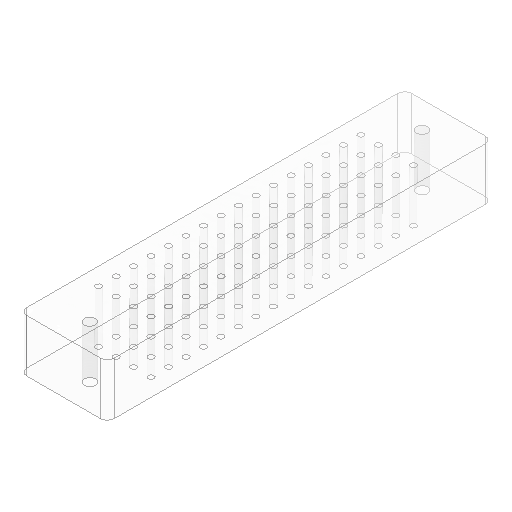
# Autodesk Inventor part: ICT-00-034
Saved by Autodesk Inventor 2026.1 (Build 301233020, 233B)
## iProperties
Company: Delta
Created: 2025-10-08
Part Number: ICT-00-034
Material: Acrílico TP
Document SubType Name: Modeling
Designer: Willian Pinheiro
Density: 1.19 g/cm^3
Appearance: Transparent - Clear
Description: Chapa T Agulha Auxiliar
Mass: 46.1991 g
Surface Area: 145.472 cm^2
Volume: 38.8228 cm^3
Dimensões: 15 x 25 x 110 mm
Total: 1
Author: Willian Pinheiro
Revision Number: 00
Title: ICT
Autodesk Inventor part; units mm, degrees
ref_plane "YZ Plane" through (0, 0, 0) normal (1, 0, 0) x (0, 1, 0)
ref_plane "XZ Plane" through (0, 0, 0) normal (0, 1, 0) x (-1, 0, 0)
ref_plane "XY Plane" through (0, 0, 0) normal (0, 0, 1) x (1, 0, 0)
sketch "Sketch1" plane through (0, 0, 0) normal (0, 0, 1) x (1, 0, 0)
  line L0 (-17.5, 0) -> (17.5, 0) construction
  line L1 (0, -77) -> (0, 77) construction
  line L2 (-12.5, 55) -> (12.5, 55)
  line L3 (12.5, 55) -> (12.5, -55)
  line L4 (12.5, -55) -> (-12.5, -55)
  line L5 (-12.5, -55) -> (-12.5, 55)
  line L6 (-7.5, -37.5) -> (7.5, -37.5) construction
  line L7 (7.5, -37.5) -> (7.5, 37.5) construction
  line L8 (7.5, 37.5) -> (-7.5, 37.5) construction
  line L9 (-7.5, 37.5) -> (-7.5, -37.5) construction
  line L10 (0, 37.5) -> (0, -37.5) construction
  circle A0 centre (0, -47.5) radius 4
  line L11 (-10.5, -40.5) -> (10.5, -40.5) construction
  line L12 (10.5, -40.5) -> (10.5, 40.5) construction
  line L13 (10.5, 40.5) -> (-10.5, 40.5) construction
  line L14 (-10.5, 40.5) -> (-10.5, -40.5) construction
  point P0 (0, 0)
  point P1 (-7.5, -32.5)
  point P2 (-7.5, -27.5)
  point P3 (-7.5, -22.5)
  point P4 (-7.5, -17.5)
  point P5 (-7.5, -12.5)
  point P6 (-7.5, -7.5)
  point P7 (-7.5, -2.5)
  point P8 (-7.5, 2.5)
  point P9 (-7.5, 7.5)
  point P10 (-7.5, 12.5)
  point P11 (-7.5, 17.5)
  point P12 (-7.5, 22.5)
  point P13 (-7.5, 27.5)
  point P14 (-7.5, 32.5)
  point P15 (-2.5, -37.5)
  point P16 (-2.5, -32.5)
  point P17 (-2.5, -27.5)
  point P18 (-2.5, -22.5)
  point P19 (-2.5, -17.5)
  point P20 (-2.5, -12.5)
  point P21 (-2.5, -7.5)
  point P22 (-2.5, -2.5)
  point P23 (-2.5, 2.5)
  point P24 (-2.5, 7.5)
  point P25 (-2.5, 12.5)
  point P26 (-2.5, 17.5)
  point P27 (-2.5, 22.5)
  point P28 (-2.5, 27.5)
  point P29 (-2.5, 32.5)
  point P30 (-2.5, 37.5)
  point P31 (2.5, -37.5)
  point P32 (2.5, -32.5)
  point P33 (2.5, -27.5)
  point P34 (2.5, -22.5)
  point P35 (2.5, -17.5)
  point P36 (2.5, -12.5)
  point P37 (2.5, -7.5)
  point P38 (2.5, -2.5)
  point P39 (2.5, 2.5)
  point P40 (2.5, 7.5)
  point P41 (2.5, 12.5)
  point P42 (2.5, 17.5)
  point P43 (2.5, 22.5)
  point P44 (2.5, 27.5)
  point P45 (2.5, 32.5)
  point P46 (2.5, 37.5)
  point P47 (7.5, -32.5)
  point P48 (7.5, -27.5)
  point P49 (7.5, -22.5)
  point P50 (7.5, -17.5)
  point P51 (7.5, -12.5)
  point P52 (7.5, -7.5)
  point P53 (7.5, -2.5)
  point P54 (7.5, 2.5)
  point P55 (7.5, 7.5)
  point P56 (7.5, 12.5)
  point P57 (7.5, 17.5)
  point P58 (7.5, 22.5)
  point P59 (7.5, 27.5)
  point P60 (7.5, 32.5)
  point P61 (0, 47.5)
  dimension "d0" = 110
  dimension "d1" = 25
  dimension "d4" = 5
  dimension "d7" = 5
  dimension "d19" = 7.5
  dimension "d20" = 8
  dimension "d21" = 3
  dimension "d22" = 81
  dimension "d23" = 21
  constraints: 26 end point, 6 parallel, 3 horizontal, 3 perpendicular, 2 midpoint, 1 centre point, 1 coincident, 1 point on line, 1 symmetric about line, 1 vertical, 70 other
  measures "d0" distance of L4.end L2.start
  measures "d1" distance of L2.start L2.end
  measures "d4" distance of L6.start point (-7.5, -32.5)
  measures "d7" distance of L6.start point (-2.5, -37.5)
  measures "d19" distance from line of L4 point (0, -47.5)
  measures "d20" diameter of A0
  measures "d21" distance between parallel lines of L14 L9
  measures "d22" distance between parallel lines of L11 L13
  measures "d23" distance between parallel lines of L12 L14
extrude "Extrusion1" add sketch "Sketch1" against normal blind 15 contours L2 L3 L4 L5 | A0
hole "Hole1" at (-7.5, -37.5, 0) at (-7.5, -32.5, 0) at (-7.5, -27.5, 0) at (-7.5, -22.5, 0) at (-7.5, -17.5, 0) at (-7.5, -12.5, 0) at (-7.5, -7.5, 0) at (-7.5, -2.5, 0) at (-7.5, 2.5, 0) at (-7.5, 7.5, 0) at (-7.5, 12.5, 0) at (-7.5, 17.5, 0) at (-7.5, 22.5, 0) at (-7.5, 27.5, 0) at (-7.5, 32.5, 0) at (-7.5, 37.5, 0) at (-2.5, -37.5, 0) at (-2.5, -32.5, 0) at (-2.5, -27.5, 0) at (-2.5, -22.5, 0) at (-2.5, -17.5, 0) at (-2.5, -12.5, 0) at (-2.5, -7.5, 0) at (-2.5, -2.5, 0) at (-2.5, 2.5, 0) at (-2.5, 7.5, 0) at (-2.5, 12.5, 0) at (-2.5, 17.5, 0) at (-2.5, 22.5, 0) at (-2.5, 27.5, 0) at (-2.5, 32.5, 0) at (-2.5, 37.5, 0) at (2.5, -37.5, 0) at (2.5, -32.5, 0) at (2.5, -27.5, 0) at (2.5, -22.5, 0) at (2.5, -17.5, 0) at (2.5, -12.5, 0) at (2.5, -7.5, 0) at (2.5, -2.5, 0) at (2.5, 2.5, 0) at (2.5, 7.5, 0) at (2.5, 12.5, 0) at (2.5, 17.5, 0) at (2.5, 22.5, 0) at (2.5, 27.5, 0) at (2.5, 32.5, 0) at (2.5, 37.5, 0) at (7.5, -37.5, 0) at (7.5, -32.5, 0) direction (0, 0, -1) diameter 1.68 end through all and at (7.5, -27.5, 0) (7.5, -22.5, 0) (7.5, -17.5, 0) (7.5, -12.5, 0) (7.5, -7.5, 0) (7.5, -2.5, 0) (7.5, 2.5, 0) (7.5, 7.5, 0) (7.5, 12.5, 0) (7.5, 17.5, 0) (7.5, 22.5, 0) (7.5, 27.5, 0) (7.5, 32.5, 0) (7.5, 37.5, 0)
hole "Hole2" at (0, 47.5, 0) at (0, -47.5, 0) direction (0, 0, -1) diameter 3.242 end through all thread size "M4x0.7" class "6H" standard "ISO Metric profile"
fillet "Fillet1" radius 2 4 edges at (-12.5, -55, -7.5) (12.5, -55, -7.5) (-12.5, 55, -7.5) (12.5, 55, -7.5)
pattern_of_nothing "Rectangular Pattern1"
equation "\"d34\" = d4"
equation "\"d37\" = d7"
body "Solid1"
